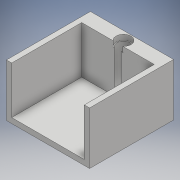
# Autodesk Inventor part: mini_holder
Saved by Autodesk Inventor 2017 (Build 210142000, 142)
## iProperties
Part Number: mini_holder
Material: Типовые
Document SubType Name: Modeling
Designer: Tolya
Density: 1 g/cm^3
Appearance: По умолчанию
Author: Tolya
Autodesk Inventor part; units mm, degrees
ref_plane "YZ Plane" through (0, 0, 0) normal (1, 0, 0) x (0, 1, 0)
ref_plane "XZ Plane" through (0, 0, 0) normal (0, 1, 0) x (-1, 0, 0)
ref_plane "XY Plane" through (0, 0, 0) normal (0, 0, 1) x (1, 0, 0)
sketch "Эскиз1" plane through (0, 0, 0) normal (0, 0, 1) x (1, 0, 0)
  arc A0 (2, -3.1721) -> (-2, -3.1721) centre (0, 0) ccw
  line L0 (-2, -3.1721) -> (2, -3.1721) construction
  line L1 (-3.75, 0) -> (-23.75, 0) construction
  line L2 (-2, -3.1721) -> (-23.75, -3.1721)
  line L3 (-23.75, -3.1721) -> (-23.75, 4.8279)
  line L4 (0, 5.092) -> (0, -4.7806)
  line L5 (2, -3.1721) -> (23.75, -3.1721)
  line L6 (23.75, -3.1721) -> (23.75, 4.8279)
  line L7 (-23.75, 4.8279) -> (23.75, 4.8279)
  point P0 (3.75, 0)
  dimension "d12" = 20
  dimension "d13" = 8
  dimension "d25" = 3.75
  constraints: 16 end point, 4 horizontal, 4 point on circle, 2 symmetric about line, 1 centre point, 1 perpendicular, 1 vertical
  measures "d12" distance of L1.start L1.end
  measures "d13" distance of L2.end L3.end
  measures "d25" radius of A0
extrude "Выдавливание1" add sketch "Эскиз1" along normal blind 30
sketch "Эскиз2" plane through (-23.75, -3.1721, 0) normal (0, -1, 0) x (1, 0, 0)
  line L0 (47.5, 0) -> (0, 0) projected
  line L1 (21.75, 0) -> (21.75, 30) projected
  line L2 (0, 0) -> (21.75, 0)
  line L3 (0, 3) -> (0, 0)
  line L4 (47.5, 0) -> (47.5, 30) projected
  line L5 (25.75, 0) -> (25.75, 30) projected
  line L6 (47.5, 0) -> (25.75, 0)
  line L7 (47.5, 3) -> (47.5, 0)
  line L8 (47.5, 30) -> (0, 30) projected
  line L9 (0, 30) -> (3, 30)
  line L10 (3, 30) -> (3, 3)
  line L11 (25.75, 30) -> (47.5, 30) projected
  line L12 (47.5, 30) -> (44.5, 30)
  line L13 (44.5, 30) -> (44.5, 3)
  line L14 (3, 3) -> (44.5, 3)
  line L15 (0, 0) -> (0, 30) projected
  line L16 (0, 30) -> (0, 0)
  line L17 (47.5, 30) -> (47.5, 0)
  point P0 (23.75, 0)
  constraints: 22 end point, 5 horizontal, 2 perpendicular, 2 vertical
extrude "Выдавливание2" add sketch "Эскиз2" along normal blind 40 contours L0 L5 L14 L13 L8 L4 | L0 L1 L14 L5 | L0 L3 L15 L8 L10 L14 L1
sketch "Эскиз3" plane through (-2, -3.1721, 3) normal (0, 0, 1) x (1, 0, 0)
  circle A0 centre (2, 3.1721) radius 3.75
  constraints: 1 centre point, 1 coincident
extrude "Выдавливание3" cut sketch "Эскиз3" along normal mid plane 40
sketch "Эскиз4" plane through (0, 0, 30) normal (0, 0, 1) x (1, 0, 0)
  circle A0 centre (0, 0) radius 4.25
  dimension "d22" = 8.5
  constraints: 1 centre point, 1 coincident
  measures "d22" diameter of A0
extrude "Выдавливание4" cut sketch "Эскиз4" against normal blind 3
